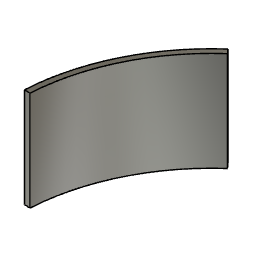
MedWise_door v1 (Autodesk Fusion 360 design; units mm, degrees)
Autodesk Fusion 360 part; units mm, degrees
sketch "Sketch1" plane through (0, 0, 0) normal (0, 0, 1) x (1, 0, 0)
  arc A0 (-45.1767, 50.8238) -> (-67.8827, 3.9931) centre (0, 0) ccw
  line L0 (0, 0) -> (-45.1767, 50.8238) construction
  line L1 (0, 0) -> (-67.8827, 3.9931) construction
  arc A1 (-46.5055, 52.3187) -> (-69.8792, 4.1105) centre (0, 0) ccw
  line L2 (0, 0) -> (-46.5055, 52.3187) construction
  line L3 (0, 0) -> (-69.8792, 4.1105) construction
  line L4 (-46.5055, 52.3187) -> (-45.1767, 50.8238)
  line L5 (-67.8827, 3.9931) -> (-69.8792, 4.1105)
  dimension "d1" = 68
  dimension "d2" = 45
  dimension "d3" = 70
  dimension "d4" = 45
  constraint coincident A0.centre L0.start
  constraint parallel L2 L4
  measures "d1" radius of A0
  measures "d2" angle of L0 L1
  measures "d3" radius of A1
  measures "d4" angle of L2 L3
extrude "Extrude1" add sketch "Sketch1" along normal blind 35
